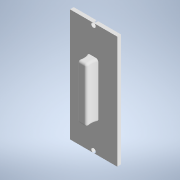
# Autodesk Inventor part: battery_case_top
Saved by Autodesk Inventor 2022 (Build 260153000, 153)
## iProperties
Created: 2022-10-11
Part Number: battery_case_top
Material: Типовые
Document SubType Name: Modeling
Designer: korsh624
Density: 1 g/cm^3
Appearance: По умолчанию
Author: korsh624
Autodesk Inventor part; units mm, degrees
ref_plane "YZ Plane" through (0, 0, 0) normal (1, 0, 0) x (0, 1, 0)
ref_plane "XZ Plane" through (0, 0, 0) normal (0, 1, 0) x (-1, 0, 0)
ref_plane "XY Plane" through (0, 0, 0) normal (0, 0, 1) x (1, 0, 0)
sketch "Эскиз1" plane through (0, 0, 0) normal (0, 0, 1) x (1, 0, 0)
  circle A0 centre (0, 98.9661) radius 2 projected
  circle A1 centre (0, -0.7112) radius 2 projected
  line L0 (-22, 101.1274) -> (22, 101.1274) projected
  line L1 (22, 101.1274) -> (22, -2.8726) projected
  line L2 (22, -2.8726) -> (-22, -2.8726) projected
  line L3 (-22, -2.8726) -> (-22, 101.1274) projected
  line L4 (21.7, 100.8274) -> (-21.7, 100.8274)
  line L5 (-21.7, 100.8274) -> (-21.7, -2.5726)
  line L6 (-21.7, -2.5726) -> (21.7, -2.5726)
  line L7 (21.7, -2.5726) -> (21.7, 100.8274)
  point P0 (0, 0)
  point P1 (-0.7318, -2.5726)
  point P2 (0.7318, -2.5726)
  point P3 (0.7318, 100.8274)
  point P4 (-0.7318, 100.8274)
  dimension "d0" = 0.3
  dimension "d1" = 0.3
  dimension "d2" = 0.3
  dimension "d3" = 0.3
  constraints: 8 end point, 2 parallel, 1 horizontal, 1 perpendicular
  measures "d0" distance between parallel lines of L4 L0
  measures "d1" distance between parallel lines of L7 L1
  measures "d2" distance between parallel lines of L6 L2
  measures "d3" distance between parallel lines of L5 L3
extrude "Выдавливание1" add sketch "Эскиз1" along normal blind 3.5 contours A0 L4 L7 L6 A1 L5
sketch "Эскиз2" plane through (0, 0, 3.5) normal (0, 0, 1) x (1, 0, 0)
  line L0 (-21.7, -2.5726) -> (-0.7318, -2.5726) projected
  arc A0 (0.7318, -2.5726) -> (-0.7318, -2.5726) centre (0, -0.7112) ccw projected
  line L1 (0.7318, -2.5726) -> (21.7, -2.5726) projected
  line L2 (21.7, -2.5726) -> (21.7, 100.8274) projected
  line L3 (21.7, 100.8274) -> (0.7318, 100.8274) projected
  arc A1 (-0.7318, 100.8274) -> (0.7318, 100.8274) centre (0, 98.9661) ccw projected
  line L4 (-0.7318, 100.8274) -> (-21.7, 100.8274) projected
  line L5 (-21.7, 100.8274) -> (-21.7, -2.5726) projected
  arc A2 (-0.7318, 100.8274) -> (0.7318, 100.8274) centre (0, 98.9661) ccw projected
  arc A3 (0.7318, -2.5726) -> (-0.7318, -2.5726) centre (0, -0.7112) ccw projected
  line L6 (0, 98.9661) -> (0, -0.7112)
  line L7 (4.3137, 74.1274) -> (-5.6863, 74.1274)
  line L8 (-5.6863, 74.1274) -> (-5.6863, 24.1274)
  line L9 (-5.6863, 24.1274) -> (4.3137, 24.1274)
  line L10 (4.3137, 24.1274) -> (4.3137, 74.1274)
  point P0 (0, 0)
  dimension "d6" = 10
  dimension "d7" = 50
  dimension "d8" = 103.4
  dimension "d9" = 26.7
  constraints: 10 end point, 2 parallel, 1 horizontal, 1 perpendicular, 1 vertical
  measures "d6" distance between parallel lines of L8 L10
  measures "d7" distance of L7.end L8.end
  measures "d8" distance between parallel lines of L1 L3
  measures "d9" distance between parallel lines of L9 L0
extrude "Выдавливание2" add sketch "Эскиз2" along normal blind 10 contours L9 L8 L7 L6 | L6 L7 L10 L9
sketch "Эскиз3" plane through (-5.6863, 74.1274, 3.5) normal (0, 1, 0) x (1, 0, 0)
  line L0 (0, 0) -> (0, -10) projected
  line L1 (4.9545, 0) -> (-16.0137, 0) projected
  arc A0 (0, -10) -> (-0.0123, 0) centre (-9.3916, -5.0116) ccw
  line L2 (10, -10) -> (0, -10) projected
  line L3 (5, -12.0906) -> (5, 6.7336) construction
  line L4 (7.6863, 0) -> (3.6863, 0) projected
  line L5 (10, 0) -> (10, -10)
  arc A1 (10.0123, 0) -> (10, -10) centre (19.3916, -5.0116) ccw
  point P0 (5.6863, 3.5)
  point P1 (6.418, 0)
  point P2 (0, -0.0232)
  point P3 (10, -0.0232)
  constraints: 4 end point, 4 point on circle, 3 symmetric about line, 2 centre point, 1 perpendicular, 1 point on line, 1 other
extrude "Выдавливание3" cut sketch "Эскиз3" against normal blind 58.75 contours A1 L5 | A0 L0
fillet "Сопряжение1" radius 2 2 edges at (4.3137, 49.1274, 13.5) (-5.6863, 49.1274, 13.5)
fillet "Сопряжение2" radius 2 10 edges at (-4.5263, 74.1274, 7.1886) (-0.6863, 74.1274, 13.5) (3.0022, 74.1274, 12.7357) (3.1537, 74.1274, 7.1886) (-4.3748, 74.1274, 12.7357) (-0.6863, 24.1274, 13.5) (3.0022, 24.1274, 12.7357) (3.1537, 24.1274, 7.1886) (-4.5263, 24.1274, 7.1886) (-4.3748, 24.1274, 12.7357)
equation "\"d0\" = d1"
equation "\"d2\" = d0"
equation "\"d3\" = d0"
equation "\"d9\" = -0.5 * d7 + 0.5 * d8"
